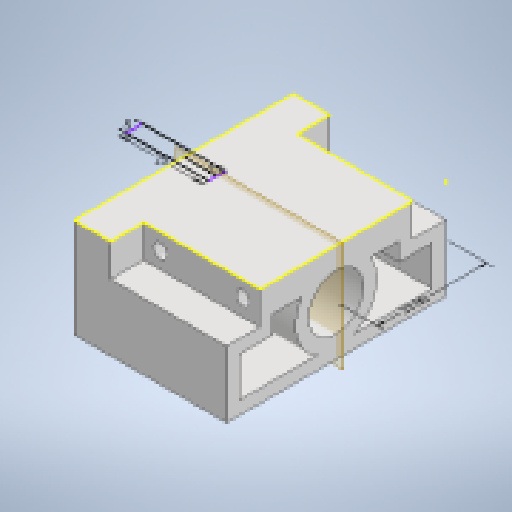
# Autodesk Inventor part: Base Catapulta
Saved by Autodesk Inventor 2024 (Build 280153000, 153)
## iProperties
Created: 2025-03-01
Part Number: Base Catapulta
Material: Genérico
Document SubType Name: Modeling
Designer: sergi
Density: 1 g/cm^3
Appearance: Valor por defecto
Author: sergi
Autodesk Inventor part; units mm, degrees
ref_plane "YZ Plane" through (0, 0, 0) normal (1, 0, 0) x (0, 1, 0)
ref_plane "XZ Plane" through (0, 0, 0) normal (0, 1, 0) x (-1, 0, 0)
ref_plane "XY Plane" through (0, 0, 0) normal (0, 0, 1) x (1, 0, 0)
sketch "Boceto1" plane through (0, 0, 0) normal (0, 1, 0) x (-1, 0, 0)
  line L0 (0, 0) -> (105, 0)
  line L1 (105, 0) -> (105, 66)
  line L2 (105, 66) -> (0, 66)
  line L3 (0, 66) -> (0, 0)
  dimension "d0" = 105
  dimension "d1" = 66
  constraints: 8 end point, 2 parallel, 1 horizontal, 1 perpendicular
  measures "d0" distance of L2.end L1.end
  measures "d1" distance of L1.end L0.end
extrude "Extrusión1" add sketch "Boceto1" along normal blind 30
sketch "Boceto2" plane through (0, 0, 66) normal (1, 0, 0) x (0, 0, -1)
  line L0 (66, 30) -> (0, 30) projected
  line L1 (0, 0) -> (66, 0) projected
  line L2 (66, 0) -> (66, 30) projected
  line L3 (0, 30) -> (66, 30) projected
  line L4 (0, 0) -> (0, 30) projected
  line L5 (66, 30) -> (0, 0)
  circle A0 centre (33, 15) radius 8.1
  dimension "d28" = 16.2
  constraints: 2 end point, 1 centre point, 1 midpoint
  measures "d28" diameter of A0
hole "Agujero1" at (0, 15, 33) direction (-1, 0, 0) diameter 16.6 depth 44
sketch "Boceto5" plane through (0, 30, 0) normal (0, 1, 0) x (1, 0, 0)
  line L0 (-105, 0) -> (-105, -66) projected
  line L1 (-105, -66) -> (0, -66) projected
  line L2 (0, -66) -> (0, 0) projected
  line L3 (0, 0) -> (-105, 0) projected
  line L4 (0, -24.7) -> (0, -41.3) projected
  line L5 (-44, -41.3) -> (-44, -24.7) projected
  line L6 (0, -41.3) -> (-44, -41.3)
  line L7 (-44, -24.7) -> (0, -24.7)
  line L8 (-46, -22.7) -> (-46, -43.3)
  line L9 (-46, -43.3) -> (2, -43.3)
  line L10 (2, -43.3) -> (2, -22.7)
  line L11 (2, -22.7) -> (-46, -22.7)
  line L12 (-46, -43.3) -> (-105, -43.3)
  line L13 (-105, 0) -> (-105, -66) projected
  line L14 (-46, -22.7) -> (-105, -22.7)
  line L15 (-105, -22.7) -> (-46, -43.3)
  line L16 (-46, -48) -> (-105, -48)
  line L17 (-105, -48) -> (-105, -18)
  line L18 (-105, -18) -> (-46, -18)
  line L19 (-46, -18) -> (-46, -48)
  line L20 (-46, -48) -> (-105, -18) construction
  line L21 (-105, -48) -> (-46, -18) construction
  point P0 (-75.5, -33)
  point P1 (-105, -18)
  dimension "d29" = 2
  dimension "d30" = 30
  constraints: 30 end point, 5 perpendicular, 4 parallel, 3 midpoint, 3 point on line, 1 horizontal, 3 other
  measures "d29" distance between parallel lines of L5 L8
  measures "d30" distance between parallel lines of L16 L18
extrude "Extrusión3" cut sketch "Boceto5" against normal through all contours L18 L19 L14 L0 | L15 L12 L0 | L14 L8 L15 | L12 L19 L16 L0
sketch "Boceto6" plane through (-46, 30, 18) normal (-1, 0, 0) x (0, 0, 1)
  circle A0 centre (20, -15) radius 1 projected
  circle A1 centre (10, -15) radius 1 projected
  point P0 (-18, -30)
hole "Agujero3" at (-46, 15, 38) at (-46, 15, 28) direction (1, 0, 0) diameter 2.2 depth 44
sketch "Boceto11" plane through (-46, 30, 18) normal (-1, 0, 0) x (0, 0, 1)
  line L0 (10, -15) -> (20, -15)
  circle A0 centre (15, -15) radius 3.35
  point P0 (-18, -30)
  dimension "d68" = 6.7
  constraints: 2 end point, 1 centre point, 1 horizontal, 1 midpoint
  measures "d68" diameter of A0
extrude "Extrusión6" cut sketch "Boceto11" against normal blind 10
sketch "Boceto12" plane through (0, 30, 0) normal (0, 1, 0) x (1, 0, 0)
  line L0 (-35, 0) -> (-35, -10) projected
  line L1 (-12.5339, -10) -> (-6, -10) projected
  line L2 (-22.4661, 0) -> (-12.5339, 0) projected
  line L3 (-35, 0) -> (0, 0) projected
  line L4 (0, -10) -> (-35, -10) projected
  line L5 (0, -66) -> (-35, -66) projected
  line L6 (-35, -56) -> (-35, -66) projected
  line L7 (-35, -56) -> (0, -56) projected
  line L8 (-46, -48) -> (-105, -48) projected
  line L9 (-105, -48) -> (-105, -66) projected
  line L10 (-105, -66) -> (0, -66) projected
  line L11 (0, -66) -> (0, 0) projected
  line L12 (0, 0) -> (-105, 0) projected
  line L13 (-105, 0) -> (-105, -18) projected
  line L14 (-105, -18) -> (-46, -18) projected
  line L15 (-46, -18) -> (-46, -48) projected
extrude "Extrusión7" cut sketch "Boceto12" against normal blind 10 contours L3 L2 L11 L4 L1 L0 | L11 L5 L6 L7
sketch "Boceto13" plane through (0, 30, 0) normal (0, 1, 0) x (1, 0, 0)
  line L0 (-35, -66) -> (-35, -56) projected
  line L1 (-35, -56) -> (0, -56) projected
  line L2 (0, -56) -> (0, -10) projected
  line L3 (0, -10) -> (-35, -10) projected
  line L4 (-35, -10) -> (-35, 0) projected
  line L5 (-35, 0) -> (-105, 0) projected
  line L6 (-105, 0) -> (-105, -18) projected
  line L7 (-105, -18) -> (-46, -18) projected
  line L8 (-46, -18) -> (-46, -48) projected
  line L9 (-46, -48) -> (-105, -48) projected
  line L10 (-105, -48) -> (-105, -66) projected
  line L11 (-105, -66) -> (-35, -66) projected
  line L12 (-105, -66) -> (-46, -66)
  line L13 (-46, -66) -> (-46, 0)
  line L14 (-46, 0) -> (-105, 0)
  line L15 (-105, 0) -> (-105, -66)
  point P0 (0, 0)
  constraints: 8 end point, 2 parallel, 1 horizontal, 1 perpendicular, 1 point on line
extrude "Extrusión8" cut sketch "Boceto13" against normal through all contours L11 L10 L9 L13 | L7 L6 L5 L13
ref_plane "Plano de trabajo4" through (-46, 0, 33) normal (0, 0, 1) x (1, 0, 0)
sketch "Boceto14" plane through (-35, 30, 56) normal (0, 0, 1) x (1, 0, 0)
  line L0 (29, 36.8) -> (29, 31.02) projected
  line L1 (29, 31.02) -> (17.6644, 31.02) projected
  line L2 (17.6644, 31.02) -> (19.7662, 36.8) projected
  line L3 (19.7662, 36.8) -> (29, 36.8) projected
  line L4 (22.4661, -4) -> (12.5339, -4) projected
  arc A0 (12.5339, -4) -> (7.2104, 2.2715) centre (5, -5) ccw projected
  line L5 (7.2104, 2.2715) -> (15.8, 25.893) projected
  line L6 (15.8, 25.893) -> (15.8, 16.82) projected
  line L7 (21.8, 10.82) -> (23, 10.82) projected
  line L8 (29, 4.82) -> (29, 2.5339) projected
  arc A1 (29, 2.5339) -> (22.4661, -4) centre (30, -5) ccw projected
  circle A2 centre (30, -5) radius 1.6 projected
  circle A3 centre (5, -5) radius 1.6 projected
  line L9 (21.8, 42.8) -> (21.8, 51) projected
  line L10 (21.8, 51) -> (30, 51) projected
  line L11 (30, 51) -> (30, 42.8) projected
  line L12 (30, 42.8) -> (21.8, 42.8) projected
  line L13 (21.8, 16.82) -> (21.8, 25.02) projected
  line L14 (21.8, 25.02) -> (30, 25.02) projected
  line L15 (30, 25.02) -> (30, 16.82) projected
  line L16 (30, 16.82) -> (21.8, 16.82) projected
  line L17 (35, 55) -> (20, 55) projected
  line L18 (20, 55) -> (0, 0) projected
  line L19 (0, 0) -> (0, -10) projected
  line L20 (35, -10) -> (0, -10) projected
  line L21 (35, 55) -> (35, -10) projected
  arc A4 (15.8, 16.82) -> (21.8, 10.82) centre (21.8, 16.82) ccw projected
  arc A5 (29, 4.82) -> (23, 10.82) centre (23, 4.82) ccw projected
  point P0 (35, -30)
hole "Agujero6" at (-30, 25, 56) at (-5, 25, 56) direction (0, 0, -1) diameter 4.2 depth 14
sketch "Boceto15" plane through (0, 30, 10) normal (0, 0, -1) x (-1, 0, 0)
  circle A0 centre (5, -5) radius 2.1 projected
  circle A1 centre (30, -5) radius 2.1 projected
  line L0 (35, 0) -> (0, 0) projected
  line L1 (35, 0) -> (35, -10) projected
  line L2 (35, -10) -> (0, -10) projected
  line L3 (0, 0) -> (0, -10) projected
  point P0 (0, -30)
hole "Agujero7" at (-5, 25, 10) at (-30, 25, 10) direction (0, 0, 1) diameter 4.2 depth 14
sketch "Boceto16" plane through (-46, 30, 0) normal (-1, 0, 0) x (0, 0, 1)
  circle A0 centre (33, -15) radius 3.35 projected
  circle A1 centre (28, -15) radius 1.1 projected
  circle A2 centre (38, -15) radius 1.1 projected
  line L0 (66, -30) -> (0, -30) projected
  line L1 (66, 0) -> (66, -30) projected
  line L2 (0, 0) -> (66, 0) projected
  line L3 (0, -30) -> (0, 0) projected
  line L4 (62, -4) -> (62, -26)
  line L5 (62, -26) -> (4, -26)
  line L6 (4, -26) -> (4, -4)
  line L7 (4, -4) -> (62, -4)
  line L8 (62, -26) -> (53.8, -26)
  line L9 (53.8, -26) -> (53.8, -17.8)
  line L10 (53.8, -17.8) -> (62, -17.8)
  line L11 (62, -17.8) -> (62, -26)
  line L12 (4, -26) -> (12.2, -26)
  line L13 (12.2, -26) -> (12.2, -17.8)
  line L14 (12.2, -17.8) -> (4, -17.8)
  line L15 (4, -17.8) -> (4, -26)
  line L16 (62, -4) -> (53.8, -4)
  line L17 (53.8, -4) -> (53.8, -12.2)
  line L18 (53.8, -12.2) -> (62, -12.2)
  line L19 (62, -12.2) -> (62, -4)
  line L20 (4, -4) -> (12.2, -4)
  line L21 (12.2, -4) -> (12.2, -12.2)
  line L22 (12.2, -12.2) -> (4, -12.2)
  line L23 (4, -12.2) -> (4, -4)
  point P0 (12.2, -4)
  point P1 (53.8, -4)
  dimension "d90" = 4
  dimension "d91" = 8.2
  dimension "d92" = 8.2
  dimension "d93" = 8.2
  dimension "d94" = 8.2
  dimension "d95" = 8.2
  dimension "d96" = 8.2
  dimension "d97" = 8.2
  dimension "d98" = 8.2
  constraints: 40 end point, 8 parallel, 4 horizontal, 4 perpendicular, 3 other
  measures "d90" distance between parallel lines of L2 L7
  measures "d91" distance of L9.end L10.end
  measures "d92" distance of L8.end L9.end
  measures "d93" distance of L14.end L13.end
  measures "d94" distance of L13.end L12.end
  measures "d95" distance of L18.end L17.end
  measures "d96" distance of L17.end L16.end
  measures "d97" distance of L21.end L22.end
  measures "d98" distance of L20.end L21.end
extrude "Extrusión9" cut sketch "Boceto16" against normal blind 10 contours L4 L18 L17 L7 | L4 L5 L9 L10 | L21 L22 L6 L7 | L5 L6 L14 L13
shell "Vaciado1" thickness 4 removed faces 1 at (0, 2.2535, 33.3335)
chamfer "Chaflán2" distance 0.5 angle 45 16 edges at (-46, 26, 8.1) (-46, 21.9, 12.2) (-46, 21.9, 4) (-46, 17.8, 8.1) (-46, 12.2, 8.1) (-46, 8.1, 4) (-46, 8.1, 12.2) (-46, 4, 8.1) (-46, 4, 57.9) (-46, 8.1, 53.8) (-46, 8.1, 62) (-46, 12.2, 57.9) (-46, 17.8, 57.9) (-46, 21.9, 53.8) (-46, 26, 57.9) (-46, 21.9, 62)
sketch "Boceto17" plane through (0, 30, 0) normal (0, 1, 0) x (1, 0, 0)
  line L0 (-46, 0) -> (-46, -66) projected
  line L1 (-35, 0) -> (-46, 0) projected
  line L2 (-46, 0) -> (-46, -66) projected
  line L3 (-46, -66) -> (-35, -66) projected
  line L4 (-35, -66) -> (-35, -56) projected
  line L5 (-35, -56) -> (0, -56) projected
  line L6 (0, -56) -> (0, -10) projected
  line L7 (0, -10) -> (-35, -10) projected
  line L8 (-35, -10) -> (-35, 0) projected
  line L9 (-35, 0) -> (-46, 0) projected
  line L10 (-46, -36.35) -> (-46, -29.65) projected
  line L11 (-56, -33) -> (-36, -33)
  line L12 (-36, -33) -> (-36, -30.5)
  line L13 (-36, -30.5) -> (-58, -30.5)
  line L14 (-58, -30.5) -> (-58, -35.5)
  line L15 (-58, -35.5) -> (-36, -35.5)
  line L16 (-36, -35.5) -> (-36, -30.5)
  line L17 (-58.2, -22) -> (-58.2, -44) projected
  line L18 (-51, -34.3366) -> (-51, -26.7075) projected
  line L19 (-56, -22) -> (-56, -44) projected
  line L20 (-51, -30.5221) -> (-56, -35.5)
  circle A0 centre (-53.5, -33.011) radius 2.5
  line L21 (-46, -33) -> (-46, -29)
  line L22 (-46, -29) -> (-36, -29)
  line L23 (-36, -29) -> (-46, -29)
  line L24 (-46, -29) -> (-46, -37)
  line L25 (-46, -37) -> (-36, -37)
  line L26 (-36, -37) -> (-36, -29)
  line L27 (-46, -37) -> (-58, -37)
  line L28 (-58, -37) -> (-58, -29)
  line L29 (-58, -29) -> (-46, -29)
  line L30 (-46, -29) -> (-46, -37)
  point P0 (0, 0)
  point P1 (-53.2654, -35.5)
  point P2 (-53.7346, -35.5)
  dimension "d105" = 22
  dimension "d106" = 5
  dimension "d107" = 5
  dimension "d111" = 4
  dimension "d112" = 10
  dimension "d113" = 8
  constraints: 34 end point, 7 parallel, 4 horizontal, 4 midpoint, 4 point on line, 3 perpendicular, 1 centre point, 1 vertical
  measures "d105" distance of L15.end L14.end
  measures "d106" distance of L14.end L13.end
  measures "d107" diameter of A0
  measures "d111" distance of L21.start L21.end
  measures "d112" distance of L21.end L22.end
  measures "d113" distance of L24.end L23.end
extrude "Extrusión10" add sketch "Boceto17" along normal blind 3 contours L22 L26 L13 L0 | L0 L13 L18 L29 | L18 L13 L19 L29 | L13 L12 L11 L0 | L0 L11 L18 L13 | L18 L20 A0 L19 L13 | L19 L13 L28 L29 | L11 L16 L15 L0 | L0 L15 A0 L18 L11 | L19 L15 L14 L13 | L18 A0 L20 | L15 L26 L25 L0 | L0 L27 L19 L15 A0 | A0 L20 L19 | L15 L19 L27 L28 | L20 A0 L15
fillet "Empalme1" radius 2.5 5 edges at (-46, 30, 33) (-41, 30, 29) (-36, 30, 36.25) (-36, 30, 29.75) (-41, 30, 37)
